Autodesk Fusion 360 part; units mm, degrees
note: some values were not read from the file. Chosen so that the rebuilt part matches the saved one: which bodies a step acts on; which face or edge a step refers to.
(part 3 of 3)
extrude "Extrude2''" cut sketch "Sketch2 (4)" against normal blind 2.38125 contours L0 L58 L59 L60 L61 | L0 L54 L55 L56 L57 | L0 L50 L51 L52 L53 | L0 L6 L7 L8 L9 | L0 L46 L47 L48 L49 | L0 L10 L11 L12 L13 | L0 L42 L43 L44 L45 | L0 L14 L15 L16 L17 | L0 L38 L39 L40 L41 | L0 L18 L19 L20 L21 | L0 L34 L35 L36 L37 | L0 L22 L23 L24 L25 | L0 L30 L31 L32 L33 | L0 L26 L27 L28 L29 picked at (38.1, 29.897917) picked at (32.971154, 31.220833) picked at (26.254808, 29.897917) picked at (-38.1, 29.897917) picked at (20.332212, 29.897917) picked at (-32.177404, 29.897917) picked at (14.409615, 29.897917) picked at (-27.048558, 31.220833) picked at (8.487019, 29.897917) picked at (-20.332212, 29.897917) picked at (2.564423, 29.897917) picked at (-15.203365, 31.220833) picked at (-3.358173, 29.897917) picked at (-8.487019, 29.897917) bodies 9 in component "rear_panel"
sketch "Sketch3 (3)" plane through (0, 171.45, 0) normal (0, 1, 0) x (-1, 0, 0) in component "rear_panel"
  line L0 (-27.842308, 28.575) -> (-27.842308, 32.54375)
  line L1 (-27.842308, 32.54375) -> (-31.383654, 32.54375)
  line L2 (-31.383654, 32.54375) -> (-31.383654, 28.575)
  line L3 (-31.383654, 28.575) -> (-33.764904, 28.575)
  line L4 (-33.764904, 28.575) -> (-33.764904, 32.54375)
  line L5 (-33.764904, 32.54375) -> (-37.30625, 32.54375)
  line L6 (-37.30625, 32.54375) -> (-37.30625, 28.575)
  line L7 (-37.30625, 28.575) -> (-39.6875, 28.575)
  line L8 (-39.6875, 28.575) -> (-39.6875, 32.54375)
  line L9 (-39.6875, 32.54375) -> (-73.2155, 32.54375)
  arc A0 (-73.2155, 32.54375) -> (-75.40625, 30.353) centre (-73.2155, 30.353) ccw
  line L10 (-75.40625, 30.353) -> (-75.40625, -30.353)
  arc A1 (-75.40625, -30.353) -> (-73.2155, -32.54375) centre (-73.2155, -30.353) ccw
  line L11 (-73.2155, -32.54375) -> (73.2155, -32.54375)
  arc A2 (73.2155, -32.54375) -> (75.40625, -30.353) centre (73.2155, -30.353) ccw
  line L12 (75.40625, -30.353) -> (75.40625, 30.353)
  arc A3 (75.40625, 30.353) -> (73.2155, 32.54375) centre (73.2155, 30.353) ccw
  line L13 (73.2155, 32.54375) -> (39.6875, 32.54375)
  line L14 (39.6875, 32.54375) -> (39.6875, 28.575)
  line L15 (39.6875, 28.575) -> (37.30625, 28.575)
  line L16 (37.30625, 28.575) -> (37.30625, 32.54375)
  line L17 (37.30625, 32.54375) -> (33.764904, 32.54375)
  line L18 (33.764904, 32.54375) -> (33.764904, 28.575)
  line L19 (33.764904, 28.575) -> (31.383654, 28.575)
  line L20 (31.383654, 28.575) -> (31.383654, 32.54375)
  line L21 (31.383654, 32.54375) -> (27.842308, 32.54375)
  line L22 (27.842308, 32.54375) -> (27.842308, 28.575)
  line L23 (27.842308, 28.575) -> (25.461058, 28.575)
  line L24 (25.461058, 28.575) -> (25.461058, 32.54375)
  line L25 (25.461058, 32.54375) -> (21.919712, 32.54375)
  line L26 (21.919712, 32.54375) -> (21.919712, 28.575)
  line L27 (21.919712, 28.575) -> (19.538462, 28.575)
  line L28 (19.538462, 28.575) -> (19.538462, 32.54375)
  line L29 (19.538462, 32.54375) -> (15.997115, 32.54375)
  line L30 (15.997115, 32.54375) -> (15.997115, 28.575)
  line L31 (15.997115, 28.575) -> (13.615865, 28.575)
  line L32 (13.615865, 28.575) -> (13.615865, 32.54375)
  line L33 (13.615865, 32.54375) -> (10.074519, 32.54375)
  line L34 (10.074519, 32.54375) -> (10.074519, 28.575)
  line L35 (10.074519, 28.575) -> (7.693269, 28.575)
  line L36 (7.693269, 28.575) -> (7.693269, 32.54375)
  line L37 (7.693269, 32.54375) -> (4.151923, 32.54375)
  line L38 (4.151923, 32.54375) -> (4.151923, 28.575)
  line L39 (4.151923, 28.575) -> (1.770673, 28.575)
  line L40 (1.770673, 28.575) -> (1.770673, 32.54375)
  line L41 (1.770673, 32.54375) -> (-1.770673, 32.54375)
  line L42 (-1.770673, 32.54375) -> (-1.770673, 28.575)
  line L43 (-1.770673, 28.575) -> (-4.151923, 28.575)
  line L44 (-4.151923, 28.575) -> (-4.151923, 32.54375)
  line L45 (-4.151923, 32.54375) -> (-7.693269, 32.54375)
  line L46 (-7.693269, 32.54375) -> (-7.693269, 28.575)
  line L47 (-7.693269, 28.575) -> (-10.074519, 28.575)
  line L48 (-10.074519, 28.575) -> (-10.074519, 32.54375)
  line L49 (-10.074519, 32.54375) -> (-13.615865, 32.54375)
  line L50 (-13.615865, 32.54375) -> (-13.615865, 28.575)
  line L51 (-13.615865, 28.575) -> (-15.997115, 28.575)
  line L52 (-15.997115, 28.575) -> (-15.997115, 32.54375)
  line L53 (-15.997115, 32.54375) -> (-19.538462, 32.54375)
  line L54 (-19.538462, 32.54375) -> (-19.538462, 28.575)
  line L55 (-19.538462, 28.575) -> (-21.919712, 28.575)
  line L56 (-21.919712, 28.575) -> (-21.919712, 32.54375)
  line L57 (-21.919712, 32.54375) -> (-25.461058, 32.54375)
  line L58 (-25.461058, 32.54375) -> (-25.461058, 28.575)
  line L59 (-25.461058, 28.575) -> (-27.842308, 28.575)
  circle A4 centre (-69.05625, -26.19375) radius 1.785938
  circle A5 centre (-69.05625, 26.19375) radius 1.785938
  circle A6 centre (69.05625, 26.19375) radius 1.785938
  circle A7 centre (69.05625, -26.19375) radius 1.785938
extrude "Extrude8''" cut sketch "Sketch3 (3)" against normal up to surface (2.38125 mm away) contours A4 | A5 | A6 | A7 picked at (-67.895552, -26.579223) picked at (-67.895552, 25.808277) picked at (70.216948, 25.808277) picked at (70.216948, -26.579223) bodies 9 in component "rear_panel"
sketch "Sketch4" plane through (0, 171.45, 0) normal (0, 1, 0) x (-1, 0, 0) in component "rear_panel"
  line L0 (-27.842308, 28.575) -> (-27.842308, 32.54375)
  line L1 (-27.842308, 32.54375) -> (-31.383654, 32.54375)
  line L2 (-31.383654, 32.54375) -> (-31.383654, 28.575)
  line L3 (-31.383654, 28.575) -> (-33.764904, 28.575)
  line L4 (-33.764904, 28.575) -> (-33.764904, 32.54375)
  line L5 (-33.764904, 32.54375) -> (-37.30625, 32.54375)
  line L6 (-37.30625, 32.54375) -> (-37.30625, 28.575)
  line L7 (-37.30625, 28.575) -> (-39.6875, 28.575)
  line L8 (-39.6875, 28.575) -> (-39.6875, 32.54375)
  line L9 (-39.6875, 32.54375) -> (-73.2155, 32.54375)
  arc A0 (-73.2155, 32.54375) -> (-75.40625, 30.353) centre (-73.2155, 30.353) ccw
  line L10 (-75.40625, 30.353) -> (-75.40625, -30.353)
  arc A1 (-75.40625, -30.353) -> (-73.2155, -32.54375) centre (-73.2155, -30.353) ccw
  line L11 (-73.2155, -32.54375) -> (73.2155, -32.54375)
  arc A2 (73.2155, -32.54375) -> (75.40625, -30.353) centre (73.2155, -30.353) ccw
  line L12 (75.40625, -30.353) -> (75.40625, 30.353)
  arc A3 (75.40625, 30.353) -> (73.2155, 32.54375) centre (73.2155, 30.353) ccw
  line L13 (73.2155, 32.54375) -> (39.6875, 32.54375)
  line L14 (39.6875, 32.54375) -> (39.6875, 28.575)
  line L15 (39.6875, 28.575) -> (37.30625, 28.575)
  line L16 (37.30625, 28.575) -> (37.30625, 32.54375)
  line L17 (37.30625, 32.54375) -> (33.764904, 32.54375)
  line L18 (33.764904, 32.54375) -> (33.764904, 28.575)
  line L19 (33.764904, 28.575) -> (31.383654, 28.575)
  line L20 (31.383654, 28.575) -> (31.383654, 32.54375)
  line L21 (31.383654, 32.54375) -> (27.842308, 32.54375)
  line L22 (27.842308, 32.54375) -> (27.842308, 28.575)
  line L23 (27.842308, 28.575) -> (25.461058, 28.575)
  line L24 (25.461058, 28.575) -> (25.461058, 32.54375)
  line L25 (25.461058, 32.54375) -> (21.919712, 32.54375)
  line L26 (21.919712, 32.54375) -> (21.919712, 28.575)
  line L27 (21.919712, 28.575) -> (19.538462, 28.575)
  line L28 (19.538462, 28.575) -> (19.538462, 32.54375)
  line L29 (19.538462, 32.54375) -> (15.997115, 32.54375)
  line L30 (15.997115, 32.54375) -> (15.997115, 28.575)
  line L31 (15.997115, 28.575) -> (13.615865, 28.575)
  line L32 (13.615865, 28.575) -> (13.615865, 32.54375)
  line L33 (13.615865, 32.54375) -> (10.074519, 32.54375)
  line L34 (10.074519, 32.54375) -> (10.074519, 28.575)
  line L35 (10.074519, 28.575) -> (7.693269, 28.575)
  line L36 (7.693269, 28.575) -> (7.693269, 32.54375)
  line L37 (7.693269, 32.54375) -> (4.151923, 32.54375)
  line L38 (4.151923, 32.54375) -> (4.151923, 28.575)
  line L39 (4.151923, 28.575) -> (1.770673, 28.575)
  line L40 (1.770673, 28.575) -> (1.770673, 32.54375)
  line L41 (1.770673, 32.54375) -> (-1.770673, 32.54375)
  line L42 (-1.770673, 32.54375) -> (-1.770673, 28.575)
  line L43 (-1.770673, 28.575) -> (-4.151923, 28.575)
  line L44 (-4.151923, 28.575) -> (-4.151923, 32.54375)
  line L45 (-4.151923, 32.54375) -> (-7.693269, 32.54375)
  line L46 (-7.693269, 32.54375) -> (-7.693269, 28.575)
  line L47 (-7.693269, 28.575) -> (-10.074519, 28.575)
  line L48 (-10.074519, 28.575) -> (-10.074519, 32.54375)
  line L49 (-10.074519, 32.54375) -> (-13.615865, 32.54375)
  line L50 (-13.615865, 32.54375) -> (-13.615865, 28.575)
  line L51 (-13.615865, 28.575) -> (-15.997115, 28.575)
  line L52 (-15.997115, 28.575) -> (-15.997115, 32.54375)
  line L53 (-15.997115, 32.54375) -> (-19.538462, 32.54375)
  line L54 (-19.538462, 32.54375) -> (-19.538462, 28.575)
  line L55 (-19.538462, 28.575) -> (-21.919712, 28.575)
  line L56 (-21.919712, 28.575) -> (-21.919712, 32.54375)
  line L57 (-21.919712, 32.54375) -> (-25.461058, 32.54375)
  line L58 (-25.461058, 32.54375) -> (-25.461058, 28.575)
  line L59 (-25.461058, 28.575) -> (-27.842308, 28.575)
  line L60 (75.40625, -0.79375) -> (-75.40625, -0.79375)
  line L61 (-75.40625, -0.79375) -> (-75.40625, 0.79375)
  line L62 (-75.40625, 0.79375) -> (75.40625, 0.79375)
  line L63 (75.40625, 0.79375) -> (75.40625, -0.79375)
  line L64 (75.40625, -0.79375) -> (-75.40625, 0.79375) construction
  line L65 (-75.40625, -0.79375) -> (75.40625, 0.79375) construction
  circle A4 centre (-69.05625, -26.19375) radius 1.785938
  circle A5 centre (69.05625, 26.19375) radius 1.785938
  circle A6 centre (-69.05625, 26.19375) radius 1.785938
  circle A7 centre (69.05625, -26.19375) radius 1.785938
  dimension "d272" = 150.8125
  dimension "d273" = 1.5875
  constraint horizontal L60
  constraint perpendicular L60 L61
  constraint parallel L60 L62
  constraint parallel L61 L63
  constraint coincident L64 origin
  constraint coincident L65 origin
extrude "Extrude4'" cut sketch "Sketch4" against normal blind 1.5875 contours L10 L12 L60 L61 L62 L63 picked at (-25.135417, 0.264583) bodies 9 in component "rear_panel"
ref_plane "WorkPlane2" through (-73.025, 93.6625, 0) normal (1, 0, 0) x (0, 0, 1) in component "rear_panel"
sketch "Sketch5 (2)" plane through (-73.025, 0, 0) normal (1, 0, 0) x (0, 1, 0) in component "rear_panel"
  line L0 (169.06875, 6.35) -> (169.06875, 3.96875)
  line L1 (169.06875, 6.35) -> (18.25625, 6.35)
  arc A0 (18.25625, 6.35) -> (15.875, 3.96875) centre (18.25625, 3.96875) ccw
  line L2 (15.875, 3.96875) -> (169.06875, 3.96875)
  line L3 (169.06875, -3.96875) -> (169.06875, -6.35)
  line L4 (169.06875, -3.96875) -> (15.875, -3.96875)
  arc A1 (15.875, -3.96875) -> (18.25625, -6.35) centre (18.25625, -3.96875) ccw
  line L5 (18.25625, -6.35) -> (169.06875, -6.35)
  line L6 (169.06875, 6.35) -> (166.6875, 6.35)
  line L7 (166.6875, 6.35) -> (166.6875, -6.35)
  line L8 (166.6875, -6.35) -> (169.06875, -6.35)
  line L9 (169.06875, -6.35) -> (169.06875, 6.35)
  dimension "d280" = 2.38125
  constraint horizontal L6
  constraint vertical L7
  constraint horizontal L8
  constraint vertical L9
extrude "Extrude6''" add sketch "Sketch5 (2)" along normal blind 146.05 contours L0 L1 L2 L6 L7 L9 | L2 L4 L7 L9 | L3 L4 L5 L7 L8 L9 picked at (168.275, 4.7625) picked at (167.48125, 1.322917) picked at (167.48125, -4.7625) bodies 9 in component "rear_panel"
fillet "Fillet1'" radius 2.38125 2 edges at (0, 166.6875, 6.35) (0, 166.6875, -6.35) on bodies 9 in component "rear_panel"
sketch "Sketch6 (2)" plane through (0, 171.45, 0) normal (0, 1, 0) x (-1, 0, 0) in component "rear_panel"
  line L0 (75.40625, -0.79375) -> (-75.40625, -0.79375)
  line L1 (-75.40625, -0.79375) -> (-75.40625, -30.353)
  arc A0 (-75.40625, -30.353) -> (-73.2155, -32.54375) centre (-73.2155, -30.353) ccw
  line L2 (-73.2155, -32.54375) -> (73.2155, -32.54375)
  arc A1 (73.2155, -32.54375) -> (75.40625, -30.353) centre (73.2155, -30.353) ccw
  line L3 (75.40625, -30.353) -> (75.40625, -0.79375)
  line L4 (0, 0) -> (0, -32.54375) construction
  line L5 (6.6675, -32.54375) -> (-6.6675, -32.54375)
  line L6 (-6.6675, -32.54375) -> (-6.6675, -18.57375)
  line L7 (-6.6675, -18.57375) -> (6.6675, -18.57375)
  line L8 (6.6675, -18.57375) -> (6.6675, -32.54375)
  line L9 (6.6675, -32.54375) -> (-6.6675, -18.57375) construction
  line L10 (-6.6675, -32.54375) -> (6.6675, -18.57375) construction
  circle A2 centre (-69.05625, -26.19375) radius 1.785938
  circle A3 centre (69.05625, -26.19375) radius 1.785938
  point P0 (0, -25.55875)
  dimension "d287" = 13.335
  dimension "d288" = 13.97
  constraint coincident L4.start origin
  constraint horizontal L5
  constraint perpendicular L5 L6
  constraint parallel L5 L7
  constraint parallel L6 L8
  constraint collinear L2 L5
extrude "Extrude7''" cut sketch "Sketch6 (2)" against normal up to surface (2.38125 mm away) contours L2 L5 L6 L7 L8 picked at (2.2225, -27.887083) bodies 9 in component "rear_panel"
ref_plane "WorkPlane1" through (0, 171.45, 0) normal (0, 1, 0) x (1, 0, 0) in component "cable_strain_relief"
sketch "Sketch1 (4)" plane through (0, 171.45, 0) normal (0, 1, 0) x (1, 0, 0) in component "cable_strain_relief"
  line L0 (-6.6675, 18.57375) -> (-6.6675, 32.54375)
  line L1 (6.6675, 18.57375) -> (-6.6675, 18.57375)
  line L2 (6.6675, 32.54375) -> (6.6675, 18.57375)
  line L3 (-73.2155, 32.54375) -> (73.2155, 32.54375)
  line L4 (6.6675, 32.54375) -> (6.6675, 30.1625) construction
  line L5 (6.6675, 30.1625) -> (-6.6675, 18.57375) construction
  line L6 (-6.35, 33.893125) -> (6.35, 33.893125)
  line L7 (9.525, 30.718125) -> (9.525, 18.018125)
  line L8 (6.35, 14.843125) -> (-6.35, 14.843125)
  line L9 (-9.525, 18.018125) -> (-9.525, 30.718125)
  line L10 (-9.525, 33.893125) -> (9.525, 14.843125) construction
  line L11 (9.525, 33.893125) -> (-9.525, 14.843125) construction
  arc A0 (6.35, 14.843125) -> (9.525, 18.018125) centre (6.35, 18.018125) ccw
  arc A1 (9.525, 30.718125) -> (6.35, 33.893125) centre (6.35, 30.718125) ccw
  arc A2 (-9.525, 18.018125) -> (-6.35, 14.843125) centre (-6.35, 18.018125) ccw
  arc A3 (-6.35, 33.893125) -> (-9.525, 30.718125) centre (-6.35, 30.718125) ccw
  circle A4 centre (0, 24.368125) radius 4.7625
  point P0 (0, 24.368125)
  dimension "d293" = 2.38125
  dimension "d294" = 19.05
  dimension "d295" = 19.05
  dimension "d296" = 3.175
  dimension "d297" = 3.175
  dimension "d298" = 3.175
  dimension "d299" = 3.175
  dimension "d300" = 9.525
  constraint perpendicular L3 L4
  constraint horizontal L6
  constraint perpendicular L6 L7
  constraint parallel L6 L8
  constraint parallel L7 L9
  constraint tangent L7 A0
  constraint tangent L8 A0
  constraint tangent L7 A1
  constraint tangent L6 A1
  constraint tangent L8 A2
  constraint tangent L9 A2
  constraint tangent L9 A3
  constraint tangent L6 A3
  measures "d296" radius of A0
  measures "d297" radius of A1
  measures "d298" radius of A2
  measures "d299" radius of A3
  measures "d300" diameter of A4
extrude "Extrude1''''" add sketch "Sketch1 (4)" along normal blind 1.5875 separate body makes body 10 in component "cable_strain_relief"
move_face "OffsetFaces1" offset 3.96875 1 faces at (-0.118634, 171.45, -32.301186) on bodies 10 in component "cable_strain_relief"
combine "Combine1'" operation cut target body 10 tool bodies 9 keep tools in component "cable_strain_relief"
combine "Combine2" operation cut target body 10 tool bodies 2 keep tools in component "cable_strain_relief"
ref_plane "WorkPlane2" through (0, 177.8, -24.368125) normal (0, 1, 0) x (1, 0, 0) in component "cable_strain_relief"
sketch "Sketch2 (5)" plane through (0, 177.8, 0) normal (0, 1, 0) x (1, 0, 0) in component "cable_strain_relief"
  circle A0 centre (0, 24.368125) radius 4.7625
sketch "Sketch3 (4)" plane through (0, 173.0375, 0) normal (0, 1, 0) x (-1, 0, 0) in component "cable_strain_relief"
  circle A0 centre (0, -24.368125) radius 4.7625
  arc A1 (-9.525, -30.718125) -> (-6.35, -33.893125) centre (-6.35, -30.718125) ccw
  line L0 (-6.35, -33.893125) -> (6.35, -33.893125)
  arc A2 (6.35, -33.893125) -> (9.525, -30.718125) centre (6.35, -30.718125) ccw
  line L1 (9.525, -30.718125) -> (9.525, -18.018125)
  arc A3 (9.525, -18.018125) -> (6.35, -14.843125) centre (6.35, -18.018125) ccw
  line L2 (6.35, -14.843125) -> (-6.35, -14.843125)
  arc A4 (-6.35, -14.843125) -> (-9.525, -18.018125) centre (-6.35, -18.018125) ccw
  line L3 (-9.525, -18.018125) -> (-9.525, -30.718125)
  circle A5 centre (0, -24.368125) radius 7.9375
  dimension "d305" = 15.875
  constraint concentric A0 A5
  measures "d305" diameter of A5
loft "Loft1" add profiles "Sketch3 (4)", "Sketch2 (5)" section 1 contours A5 picked at (6.831884, -24.999071) section 2 bodies 10 in component "cable_strain_relief"
ref_plane "WorkPlane4" through (0, 170.259375, -24.368125) normal (0, -1, 0) x (-1, 0, 0) in component "cable_strain_relief"
mirror "Mirror1" about plane through (0, 170.259375, -24.368125) normal (0, -1, 0) of "Loft1" in component "cable_strain_relief"
sketch "Sketch5 (3)" plane through (0, 177.8, 0) normal (0, 1, 0) x (-1, 0, 0) in component "cable_strain_relief"
  circle A0 centre (0, -24.368125) radius 4.7625
  circle A1 centre (0, -24.368125) radius 4.7625
  constraint concentric A0 A1
extrude "Extrude2'''" cut sketch "Sketch5 (3)" against normal up to surface (15.08125 mm away) bodies 10 in component "cable_strain_relief"
ref_plane "WorkPlane5" through (0, 170.259375, -24.368125) normal (0, 0, 1) x (1, 0, 0) in component "cable_strain_relief"
split "Split1" by plane through (0, 170.259375, -24.368125) normal (0, 0, 1) bodies 10 makes body 11 at (6.496837, 165.364583, -23.747752) in component "cable_strain_relief"
sketch "Sketch22" plane through (76.2, 0, 0) normal (1, 0, 0) x (0, 1, 0) in component "enclosure"
  line L0 (1.5875, 0.79375) -> (1.5875, -0.79375)
  line L1 (1.5875, -0.79375) -> (171.45, -0.79375)
  line L2 (171.45, -0.79375) -> (171.45, 0.79375)
  line L3 (171.45, 0.79375) -> (1.5875, 0.79375)
  line L4 (169.8625, 0.79375) -> (169.8625, -0.79375)
  line L5 (169.8625, -0.79375) -> (169.8625, 0.79375)
  line L6 (169.8625, 0.79375) -> (171.45, 0.79375)
  line L7 (171.45, 0.79375) -> (171.45, -0.79375)
  line L8 (171.45, -0.79375) -> (169.8625, -0.79375)
  line L9 (169.8625, -0.79375) -> (169.8625, 0.79375)
  constraint horizontal L6
  constraint vertical L7
  constraint horizontal L8
  constraint vertical L9
extrude "Extrude17" cut sketch "Sketch22" against normal up to surface (152.4 mm away) contours L1 L2 L3 L4 L5 L6 L7 L8 L9 picked at (170.391667, 0.264583) bodies 2 in component "enclosure"
sketch "Sketch23" plane through (50.389094, 0, 0) normal (1, 0, 0) x (0, 1, 0) in component "enclosure"
  line L0 (-7.9375, 30.95625) -> (-5.55625, 28.575)
  line L1 (-5.55625, 28.575) -> (1.5875, 28.575)
  line L2 (1.5875, 28.575) -> (1.5875, 30.95625)
  line L3 (1.5875, 30.95625) -> (0, 30.95625)
  line L4 (0, 30.95625) -> (-1.586896, 32.515688)
  line L5 (-1.586896, 32.515688) -> (-7.9375, 32.404838)
  line L6 (-7.9375, 32.404838) -> (-7.9375, 30.95625)
  line L7 (0, 0) -> (-23.643409, 0) construction
  line L8 (-1.586896, 32.515688) -> (-7.9375, 30.95625)
  line L9 (-7.9375, 30.95625) -> (-7.9375, 32.404838)
  line L10 (-7.9375, 32.404838) -> (-1.586896, 32.515688)
  line L11 (-7.9375, -30.95625) -> (-7.9375, -32.404838)
  line L12 (-7.9375, -32.404838) -> (-1.586896, -32.515688)
  line L13 (-1.586896, -32.515688) -> (-7.9375, -30.95625)
  constraint coincident L7.start origin
  constraint horizontal L7
extrude "Extrude18" cut sketch "Sketch23" against normal up to surface (100.778188 mm away) contours L5 L6 L8 L9 L10 | L11 L12 L13 picked at (-5.820632, 31.958925) picked at (-5.820632, -31.958925) bodies 2 in component "enclosure"
sketch "Sketch24" plane through (0, 0, 12.7) normal (0, 0, 1) x (-1, 0, 0) in component "enclosure"
  line L0 (-71.4375, 5.55625) -> (-73.81875, 7.9375)
  line L1 (-73.81875, 7.9375) -> (-75.267338, 7.9375)
  line L2 (-75.267338, 7.9375) -> (-75.378188, 1.586896)
  line L3 (-75.378188, 1.586896) -> (-73.81875, 0)
  line L4 (-73.81875, 0) -> (-73.81875, -1.5875)
  line L5 (-73.81875, -1.5875) -> (-71.4375, -1.5875)
  line L6 (-71.4375, -1.5875) -> (-71.4375, 5.55625)
  line L7 (0, 0) -> (0, 31.510835) construction
  line L8 (-75.378188, 1.586896) -> (-73.81875, 7.9375)
  line L9 (-75.378188, 1.586896) -> (-75.267338, 7.9375)
  line L10 (-75.267338, 7.9375) -> (-73.81875, 7.9375)
  line L11 (75.378188, 1.586896) -> (73.81875, 7.9375)
  line L12 (75.378188, 1.586896) -> (75.267338, 7.9375)
  line L13 (75.267338, 7.9375) -> (73.81875, 7.9375)
  constraint coincident L7.start origin
  constraint vertical L7
extrude "Extrude19" cut sketch "Sketch24" against normal up to surface (25.4 mm away) contours L1 L2 L8 L9 L10 | L11 L12 L13 picked at (-74.821425, 5.820632) picked at (74.821425, 5.820632) bodies 2 in component "enclosure"
extrude "Extrude3'" cut 1 faces at (2.116667, 169.06875, -17.330208) along direction (0, -1, 0) blind 0.396875 on bodies 11 bodies 11 in component "cable_strain_relief"
extrude "Extrude4''" cut 1 faces at (-7.62, 169.06875, -29.21) along direction (0, -1, 0) blind 0.396875 on bodies 10 bodies 10 in component "cable_strain_relief"
extrude "Extrude5'" cut 1 faces at (7.62, 169.06875, -29.21) along direction (0, -1, 0) blind 0.396875 on bodies 10 bodies 10 in component "cable_strain_relief"
ref_plane "WorkPlane6" through (0, 169.465625, -32.54375) normal (0, 0, -1) x (1, 0, 0) in component "cable_strain_relief"
sketch "Sketch6 (3)" plane through (0, 0, -32.54375) normal (0, 0, -1) x (-1, 0, 0) in component "cable_strain_relief"
  line L0 (-9.525, 168.671875) -> (-9.525, 167.48125)
  line L1 (-9.525, 167.48125) -> (-9.525, 168.671875)
  line L2 (9.525, 168.671875) -> (9.525, 167.48125)
  line L3 (9.525, 167.48125) -> (9.525, 168.671875)
  line L4 (9.525, 168.671875) -> (9.525, 173.805888) construction
  line L5 (-9.525, 168.671875) -> (-9.525, 174.120625) construction
  line L6 (6.6675, 171.45) -> (-6.6675, 171.45) construction
  line L7 (9.525, 171.45) -> (-9.525, 171.39625) construction
  line L8 (9.525, 171.45) -> (-9.525, 171.45)
  line L9 (-9.525, 171.45) -> (-9.525, 159.327998)
  line L10 (-9.525, 159.327998) -> (9.525, 159.327998)
  line L11 (9.525, 159.327998) -> (9.525, 171.45)
  constraint parallel L3 L4
  constraint parallel L0 L5
  constraint coincident L4 L7.start
  constraint horizontal L8
  constraint vertical L9
  constraint horizontal L10
  constraint vertical L11
extrude "Extrude6'''" cut sketch "Sketch6 (3)" against normal blind 0.79375 bodies 10 in component "cable_strain_relief"
ref_plane "WorkPlane9" through (71.4375, -17.859375, -16.336231) normal (-1, 0, 0) x (0, 0, 1) in component "face"
sketch "Sketch20" plane through (71.4375, 0, 0) normal (-1, 0, 0) x (0, -1, 0) in component "face"
  line L0 (16.66875, -17.526856) -> (19.05, -17.526856) construction
  line L1 (19.05, -17.526856) -> (16.66875, -17.526856) construction
  line L2 (16.66875, -15.145606) -> (19.05, -15.145606) construction
  line L3 (19.05, -15.145606) -> (16.66875, -15.145606) construction
  line L4 (16.66875, 21.054976) -> (16.66875, 23.436226) construction
  line L5 (16.66875, 23.436226) -> (16.66875, 21.054976) construction
  line L6 (16.66875, -17.526856) -> (16.66875, -15.145606) construction
  line L7 (16.66875, -15.145606) -> (16.66875, -17.526856) construction
  line L8 (16.66875, -30.062017) -> (16.66875, -32.252433) construction
  line L9 (16.66875, -30.062017) -> (16.66875, 30.062017) construction
  line L10 (16.66875, 32.252433) -> (16.66875, 30.062017) construction
  line L11 (16.66875, 32.252433) -> (16.66875, 30.062017) construction
  line L12 (16.66875, 30.062017) -> (16.66875, -30.062017) construction
  line L13 (16.66875, -30.062017) -> (16.66875, -32.252433) construction
  line L14 (16.66875, -3.948149) -> (16.66875, -6.329399) construction
  line L15 (16.66875, -6.329399) -> (16.66875, -3.948149) construction
  line L16 (16.66875, 20.261226) -> (16.66875, -3.154399) construction
  line L17 (16.66875, -3.154399) -> (16.66875, 20.261226) construction
  line L18 (16.66875, 13.954981) -> (16.66875, 29.829981) construction
  line L19 (16.66875, 29.829981) -> (16.66875, 13.954981) construction
  line L20 (19.05, 28.242481) -> (19.05, 15.542481) construction
  line L21 (19.05, 15.542481) -> (19.05, 28.242481) construction
  line L22 (19.05, -5.535649) -> (19.05, 22.642476) construction
  line L23 (19.05, 22.642476) -> (19.05, -5.535649) construction
  line L24 (19.05, -15.145606) -> (19.05, -17.526856) construction
  line L25 (19.05, -17.526856) -> (19.05, -15.145606) construction
  line L26 (19.05, -30.021177) -> (19.05, -34.592481) construction
  line L27 (19.05, -30.021177) -> (19.05, -34.592481) construction
  line L28 (19.05, -30.021177) -> (19.05, 30.021177) construction
  line L29 (19.05, 34.592481) -> (19.05, 30.021177) construction
  line L30 (19.05, 34.592481) -> (19.05, 30.021177) construction
  line L31 (19.05, 30.021177) -> (19.05, -30.021177) construction
  line L32 (19.05, -15.145606) -> (17.4625, -15.145606)
  line L33 (17.4625, -15.145606) -> (16.66875, -15.145606)
  line L34 (16.66875, -15.145606) -> (16.66875, -17.526856)
  line L35 (16.66875, -17.526856) -> (17.4625, -17.526856)
  line L36 (17.4625, -17.526856) -> (17.4625, -15.145606)
  line L37 (19.05, -15.145606) -> (19.05, -17.526856) construction
  line L38 (19.05, -16.336231) -> (16.66875, -16.336231) construction
  line L39 (16.66875, -15.145606) -> (16.66875, -12.764356) construction
  line L40 (16.66875, -17.526856) -> (16.66875, -19.908106) construction
  line L41 (16.66875, -12.764356) -> (14.2875, -12.764356)
  line L42 (14.2875, -12.764356) -> (14.2875, -19.908106)
  line L43 (14.2875, -19.908106) -> (16.66875, -19.908106)
  line L44 (16.66875, -19.908106) -> (16.66875, -12.764356)
  dimension "d329" = 1.5875
  dimension "d330" = 2.38125
  dimension "d331" = 2.38125
  dimension "d332" = 2.38125
  constraint perpendicular L6 L32
  constraint horizontal L33
  constraint vertical L34
  constraint horizontal L35
  constraint vertical L36
  constraint perpendicular L33 L39
  constraint perpendicular L0 L40
  constraint horizontal L41
  constraint vertical L42
  constraint horizontal L43
  constraint vertical L44
extrude "Extrude15'" add sketch "Sketch20" along normal up to surface (142.875 mm away) contours L33 L34 L35 L36 L44 picked at (16.933333, -15.939356) bodies 1 in component "face"
extrude "Extrude16'" add sketch "Sketch20" along normal up to surface contours L34 L41 L42 L43 L44 picked at (15.08125, -16.733106) end surface through (75.406613, 0.041559, 34.925) normal (-0.9998477, 0.01745241, 0) offset 0 bodies 1 in component "face"
extrude "Extrude17'" add sketch "Sketch20" along normal up to surface contours L34 L41 L42 L43 L44 picked at (15.08125, -16.733106) end surface through (-75.406613, 0.041559, -34.925) normal (0.9998477, 0.01745241, 0) offset 0 bodies 1 in component "face"
component "face" placed x (1, 0, 0) y (0, 1, 0) z (0, 0, 1) at (0, 0, 0)
component "enclosure" placed x (1, 0, 0) y (0, 1, 0) z (0, 0, 1) at (0, 0, 0)
component "badge" placed x (1, 0, 0) y (0, 1, 0) z (0, 0, 1) at (0, 0, 0)
component "rear_panel" placed x (1, 0, 0) y (0, 1, 0) z (0, 0, 1) at (0, 0, 0)
component "cable_strain_relief" placed x (1, 0, 0) y (0, 1, 0) z (0, 0, 1) at (0, 0, 0)
equation "accent_line_bottom_offset = 43/64\"" comment "Face accent line distance from bottom"
equation "accent_line_height = 3/32\"" comment "Face accent line height"
equation "accent_line_width = enclosure_width - 1/2\"" comment "Face accent line height"
equation "enclosure_corner_radius = 0.18 in" comment "Corner radius for enclosure"
equation "enclosure_depth = 8 1/2\" - 1 in" comment "Overall enclosure depth"
equation "enclosure_height = 2 3/4\"" comment "Overall enclosure height"
equation "enclosure_width = 6 1/8\"" comment "Overall enclosure width"
equation "face_depth = 3/4\"" comment "Face component depth"
equation "face_extrude_angle = 1 deg" comment "Face component extrude angle"
equation "gotek_mount_sleeve_depth = 1 1/2\"" comment "Gotek drive mounting sleeve depth"
equation "gotek_mount_sleeve_face_depth = 7/64\"" comment "Gotek drive face depth used to lock into mounting sleeve"
equation "gotek_mount_sleeve_height = 63/64\"" comment "Gotek drive mounting sleeve height"
equation "gotek_mount_sleeve_latch_height = 49/64\"" comment "Gotek drive mounting sleeve latch height"
equation "gotek_mount_sleeve_latch_width = 3/64\"" comment "Gotek drive mounting sleeve latch width"
equation "gotek_mount_sleeve_width = 4.02 in" comment "Gotek drive mounting sleeve width"
equation "shell_thickness = 3/32\"" comment "Overall enclosure shell thickness"
equation "d29 = enclosure_width"
equation "d30 = enclosure_height"
equation "d31 = -face_depth"
equation "d32 = -face_extrude_angle"
equation "d34 = enclosure_corner_radius"
equation "d35 = shell_thickness"
equation "d36 = accent_line_width"
equation "d37 = accent_line_height"
equation "d38 = accent_line_bottom_offset"
equation "d39 = 0\""
equation "accent_line_depth = 1/16\""
equation "d42 = gotek_mount_sleeve_width + ( shell_thickness * 2 )"
equation "d43 = gotek_mount_sleeve_height + ( shell_thickness * 2 )"
equation "d44 = gotek_mount_sleeve_depth"
equation "d46 = shell_thickness"
equation "d59 = 0\""
equation "d60 = gotek_mount_sleeve_face_depth"
equation "d61 = 0\""
equation "d63 = 0\""
equation "d64 = gotek_mount_sleeve_latch_width"
equation "d65 = 0\""
equation "d67 = 0\""
equation "d68 = gotek_mount_sleeve_latch_height"
equation "d69 = 0\""
equation "gotek_mounting_sleeve_latch_bottom_gap_height = 1/32\""
equation "gotek_mounting_sleeve_latch_bottom_gap_depth = gotek_mount_sleeve_depth * 0.5"
equation "d73 = gotek_mounting_sleeve_latch_bottom_gap_depth"
equation "d74 = gotek_mounting_sleeve_latch_bottom_gap_height"
equation "d75 = 0\""
equation "gotek_window_inset = 1/32\""
equation "d80 = 0\""
equation "d81 = gotek_window_inset"
equation "d82 = 0\""
equation "d84 = 0\""
equation "face_seam_inset = 1/16\"" comment "The inset of the seam between the face and the enclsoure body"
equation "face_seam_depth = 1/16\"" comment "The depth of the seam between the face and the enclosure body"
equation "d97 = -face_seam_inset"
equation "d98 = -( shell_thickness + face_seam_inset )"
equation "d99 = face_seam_depth"
equation "accent_line_filler_inset = 0.002 in"
equation "accent_line_back_offset = shell_thickness / 2"
equation "accent_line_filler_depth = shell_thickness - 1/16\""
equation "d117 = shell_thickness"
equation "enclosure_face_clip_depth = 3/8\""
equation "d119 = -enclosure_face_clip_depth"
equation "enclosure_face_clip_size = 1 in"
equation "d131 = enclosure_face_clip_size"
equation "d132 = enclosure_face_clip_size"
equation "d133 = 0\""
equation "d135 = 0\""
equation "d137 = shell_thickness"
equation "d138 = enclosure_corner_radius"
equation "d139 = enclosure_corner_radius"
equation "d140 = enclosure_corner_radius"
equation "d141 = enclosure_corner_radius"
equation "d142 = enclosure_depth - face_depth - face_seam_depth"
equation "d144 = -shell_thickness"
equation "d155 = shell_thickness"
equation "d156 = shell_thickness"
equation "d157 = shell_thickness"
equation "d158 = 0\""
equation "d160 = face_seam_inset"
equation "d161 = face_seam_inset"
equation "d162 = 0\""
equation "d164 = -shell_thickness"
equation "d166 = 0\""
equation "d167 = 3/4\""
equation "rear_screw_insert_diameter = 9/64\""
equation "rear_screw_support_size = 1/2\""
equation "rear_screw_insert_depth = 3/8\""
equation "rear_screw_hole_diameter = 9/64\""
equation "d172 = rear_screw_support_size"
equation "d173 = rear_screw_support_size"
equation "d174 = rear_screw_insert_diameter"
equation "d175 = -rear_screw_support_size"
equation "d177 = rear_screw_hole_diameter"
equation "d178 = -rear_screw_insert_depth"
equation "badge_offset = 1/4\""
equation "badge_size = 1/2\""
equation "d182 = badge_size"
equation "d183 = badge_size"
equation "d184 = badge_offset"
equation "d185 = badge_offset"
equation "badge_depth = 1/16\""
equation "d187 = -badge_depth"
equation "d189 = badge_size"
equation "d190 = badge_size"
equation "d191 = badge_depth"
equation "d193 = badge_depth"
equation "d194 = 0\""
equation "d195 = badge_size"
equation "d196 = badge_size"
equation "d197 = badge_depth"
equation "badge_logo_depth = 1/64\""
equation "d200 = badge_logo_depth"
equation "foot_pad_size = 3/4\""
equation "foot_pad_offset = 3/4\""
equation "foot_pad_front_offset = 1/4\""
equation "d205 = foot_pad_size"
equation "d206 = foot_pad_size"
equation "d207 = foot_pad_offset"
equation "d208 = foot_pad_front_offset"
equation "d209 = foot_pad_size"
equation "d210 = foot_pad_size"
equation "d211 = foot_pad_offset"
equation "d212 = foot_pad_offset"
equation "foot_pad_recess = 1/32\""
equation "d214 = -foot_pad_recess"
equation "bottom_front_grill_depth = 1/2\""
equation "bottom_front_grill_width = 1/16\""
equation "bottom_front_grill_count = 11"
equation "d223 = bottom_front_grill_width"
equation "d224 = bottom_front_grill_depth"
equation "d225 = bottom_front_grill_count"
equation "d227 = 1 29/64\""
equation "d228 = 0\""
equation "d229 = 0\""
equation "bottom_label_depth = 3 in"
equation "bottom_label_width = 2 in"
equation "d233 = bottom_label_width"
equation "d234 = bottom_label_depth"
equation "d235 = -foot_pad_recess"
equation "top_rear_grill_inset = 1.5 in"
equation "top_rear_grill_count = 14"
equation "top_rear_grill_depth = 1/4\""
equation "top_rear_grill_width = 3/32\""
equation "d249 = top_rear_grill_inset"
equation "d250 = top_rear_grill_inset"
equation "d251 = top_rear_grill_width"
equation "d252 = top_rear_grill_depth"
equation "d253 = top_rear_grill_count"
equation "d255 = -( enclosure_width - ( 2 * top_rear_grill_inset ) - top_rear_grill_width )"
equation "d256 = 0\""
equation "d257 = 0\""
equation "d259 = 0\""
equation "d260 = shell_thickness"
equation "d262 = top_rear_grill_width"
equation "d263 = top_rear_grill_depth - shell_thickness"
equation "d264 = top_rear_grill_count"
equation "d266 = enclosure_width - ( 2 * top_rear_grill_inset ) - top_rear_grill_width"
equation "d267 = 0\""
equation "d268 = -shell_thickness"
equation "d272 = enclosure_width - ( 2 * shell_thickness )"
equation "d273 = face_seam_depth"
equation "d274 = -face_seam_inset"
equation "d276 = 0\""
equation "d280 = shell_thickness"
equation "d281 = enclosure_width - ( 4 * shell_thickness )"
equation "d284 = shell_thickness"
equation "cable_diameter = 3/8\""
equation "rear_panel_cable_port_size = 1/2\""
equation "d287 = rear_panel_cable_port_size * 1.05"
equation "d288 = rear_panel_cable_port_size * 1.1"
equation "d289 = 0\""
equation "d291 = 0\""
equation "cable_strain_relief_size = rear_panel_cable_port_size + 1/4\""
equation "d293 = shell_thickness"
equation "d294 = cable_strain_relief_size"
equation "d295 = cable_strain_relief_size"
equation "d296 = 1/8\""
equation "d297 = 1/8\""
equation "d298 = 1/8\""
equation "d299 = 1/8\""
equation "d300 = cable_diameter"
equation "d301 = 1/16\""
equation "d303 = shell_thickness + 1/16\""
equation "d304 = shell_thickness * 2"
equation "d305 = cable_diameter + ( 1/4\" )"
equation "d308 = 1/128\""
equation "d309 = 0\""
equation "d311 = 0\""
equation "d313 = 0\""
equation "d315 = 0\""
equation "d317 = 0\""
equation "d319 = -1/64\""
equation "d321 = -1/64\""
equation "d323 = -1/64\""
equation "d325 = 0\""
equation "d326 = -1/32\""
equation "d328 = 0\""
equation "d329 = face_seam_depth"
equation "d330 = shell_thickness"
equation "d331 = shell_thickness"
equation "d332 = shell_thickness"
equation "d333 = 0\""
equation "d335 = 0\""
equation "d337 = 0\""
named bodies: "face", "bottom", "top"
